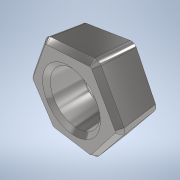
# Autodesk Inventor part: Гайка М5
Saved by Autodesk Inventor 2021.1 (Build 251245010, 245A)
## iProperties
Created: 2025-12-08
Part Number: Гайка М5
Material: Типовые
Document SubType Name: Modeling
Designer: Андрей Тарасов
Density: 1 g/cm^3
Appearance: По умолчанию
Author: Андрей Тарасов
Autodesk Inventor part; units mm, degrees
ref_plane "YZ Plane" through (0, 0, 0) normal (1, 0, 0) x (0, 1, 0)
ref_plane "XZ Plane" through (0, 0, 0) normal (0, 1, 0) x (-1, 0, 0)
ref_plane "XY Plane" through (0, 0, 0) normal (0, 0, 1) x (1, 0, 0)
sketch "Эскиз1" plane through (0, 0, 0) normal (0, 0, 1) x (1, 0, 0)
  circle A0 centre (0, 0) radius 2.5
  line L0 (2.3094, 4) -> (4.6188, 0)
  line L1 (4.6188, 0) -> (2.3094, -4)
  line L2 (2.3094, -4) -> (-2.3094, -4)
  line L3 (-2.3094, -4) -> (-4.6188, 0)
  line L4 (-4.6188, 0) -> (-2.3094, 4)
  line L5 (-2.3094, 4) -> (2.3094, 4)
  dimension "d0" = 5
  dimension "d1" = 8
  constraints: 12 end point, 2 coincident, 1 centre point, 1 horizontal, 13 other
  measures "d0" diameter of A0
  measures "d1" distance between parallel lines of L5 L2
extrude "Выдавливание1" add sketch "Эскиз1" along normal blind 4
fillet "Сопряжение1" radius 0.6 6 edges at (-4.6188, 0, 2) (-2.3094, -4, 2) (2.3094, -4, 2) (4.6188, 0, 2) (2.3094, 4, 2) (-2.3094, 4, 2)
chamfer "Фаска1" distance 0.4 angle 45 26 edges at (0, 4, 0) (-2.263, 3.9196, 0) (-3.4641, 2, 0) (-4.526, 0, 0) (-3.4641, -2, 0) (-2.263, -3.9196, 0) (0, -4, 0) (2.263, -3.9196, 0) (3.4641, -2, 0) (4.526, 0, 0) (3.4641, 2, 0) (2.263, 3.9196, 0) (0, 4, 4) (-2.263, 3.9196, 4) (-3.4641, 2, 4) (-4.526, 0, 4) (-3.4641, -2, 4) (-2.263, -3.9196, 4) (0, -4, 4) (2.263, -3.9196, 4) (3.4641, -2, 4) (4.526, 0, 4) (3.4641, 2, 4) (2.263, 3.9196, 4) (-2.5, 0, 4) (-2.5, 0, 0)
